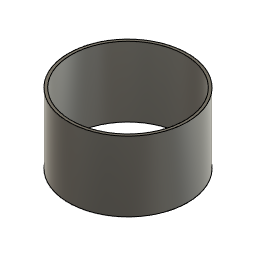
Cuvette holder storage v3 (Autodesk Fusion 360 design; units mm, degrees)
Autodesk Fusion 360 part; units mm, degrees
sketch "Sketch1" plane through (0, 0, 0) normal (0, 1, 0) x (1, 0, 0)
  circle A0 centre (0, 0) radius 51
  circle A1 centre (0, 0) radius 48.75
  circle A2 centre (0, 0) radius 38
  dimension "d1" = 102
  dimension "d2" = 97.5
  dimension "d3" = 76
  constraint coincident A0.centre A1.centre
  constraint concentric A0 A1
  measures "d1" diameter of A0
  measures "d2" diameter of A1
  measures "d3" diameter of A2
extrude "Extrude1" add sketch "Sketch1" along normal blind 2 contours A0 | A1 | A2
extrude "Extrude2" add sketch "Sketch1" against normal blind 15 contours A1
extrude "Extrude3" add sketch "Sketch1" against normal blind 58 contours A0
extrude "Extrude4" cut 1 faces at (44.8437, -15, 4.3098) along direction (0, 1, 0) up to surface (15 mm away)
extrude "Extrude5" cut sketch "Sketch1" along normal blind 20 contours A1 | A2
